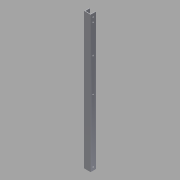
# Autodesk Inventor part: 26in C-Channel Right
Saved by Autodesk Inventor 2013 (Build 170138000, 138)
## iProperties
Created: 2013-01-08
Part Number: 26in C-Channel Right
Material: Aluminum 6061
Document SubType Name: Modeling
Designer: Naphat
Density: 1 g/cm^3
Author: Naphat
Autodesk Inventor part; units mm, degrees
ref_plane "YZ Plane" through (0, 0, 0) normal (1, 0, 0) x (0, 1, 0)
ref_plane "XZ Plane" through (0, 0, 0) normal (0, 1, 0) x (-1, 0, 0)
ref_plane "XY Plane" through (0, 0, 0) normal (0, 0, 1) x (1, 0, 0)
sketch "Sketch1" plane through (0, 0, 0) normal (0, 0, 1) x (1, 0, 0)
  line L0 (-15.7, 12.7) -> (-12.7, 12.7)
  line L1 (-12.7, 12.7) -> (-12.7, -9.7)
  line L2 (-12.7, -9.7) -> (12.7, -9.7)
  line L3 (12.7, -9.7) -> (12.7, 12.7)
  line L4 (12.7, 12.7) -> (15.7, 12.7)
  line L5 (15.7, 12.7) -> (15.7, -12.7)
  line L6 (15.7, -12.7) -> (-15.7, -12.7)
  line L7 (-15.7, -12.7) -> (-15.7, 12.7)
  point P0 (0, 0)
  dimension "d0" = 3
  dimension "d2" = 3
  dimension "d3" = 25.4
  dimension "d4" = 31.4
  dimension "d5" = 15.7
  dimension "d7" = 12.7
  dimension "d8" = 3
  constraints: 16 end point, 5 parallel, 1 collinear, 1 horizontal, 1 perpendicular
  measures "d0" distance of L0.start L0.end
  measures "d2" distance of L3.end L4.end
  measures "d3" distance of L6.end L0.start
  measures "d4" distance of L5.end L6.end
  measures "d5" distance from line of point (0, 0) L7
  measures "d7" distance from line of L6 point (0, 0)
  measures "d8" distance between parallel lines of L6 L2
extrude "Extrusion1" add sketch "Sketch1" against normal blind 660.4
sketch "Sketch5" plane through (15.7, -12.7, 0) normal (1, 0, 0) x (0, 0, -1)
  circle A0 centre (16, 12.7) radius 3.175
  circle A1 centre (644.4, 12.7) radius 3.175
  line L0 (0, 25.4) -> (0, 0) projected
  line L1 (660.4, 25.4) -> (660.4, 0) projected
  line L2 (0, 25.4) -> (660.4, 25.4) projected
  point P0 (0, 12.7)
  dimension "d56" = 6.35
  dimension "d65" = 6.35
  dimension "d70" = 16
  dimension "d71" = 25.4
  dimension "d72" = 12.7
  dimension "d73" = 16
  constraints: 2 centre point, 1 horizontal alignment
  measures "d56" diameter of A0
  measures "d65" diameter of A1
  measures "d70" distance from line of A1.centre L1
  measures "d71" distance of L1.start L1.end
  measures "d72" distance from line of L2 A1.centre
  measures "d73" distance from line of L0 A0.centre
extrude "Extrusion5" cut sketch "Sketch5" against normal blind 76.2
sketch "Sketch6" plane through (-15.7, -12.7, 0) normal (-1, 0, 0) x (0, 0, 1)
  circle A0 centre (-37.4708, 12.3) radius 3.175
  circle A1 centre (-177.8, 12.3) radius 3.175
  circle A2 centre (-340.3166, 12.3) radius 3.175
  point P0 (0, 12.7)
  constraints: 3 centre point
extrude "Extrusion6" cut sketch "Sketch6" against normal blind 50.8
equation "\"d2\" = d0"
equation "\"d5\" = 0.5 * d4"
equation "\"d7\" = 0.5 * d3"
equation "\"d8\" = d0"
equation "\"d65\" = d64"
equation "\"d72\" = 0.5 * d71"
equation "\"d73\" = d70"
equation "\"d58\" = d56"
equation "\"d59\" = d58"
equation "\"d60\" = d59"
equation "\"d61\" = d60"
equation "\"d62\" = d61"
equation "\"d63\" = d62"
equation "\"d64\" = d63"
body "Solid1"
